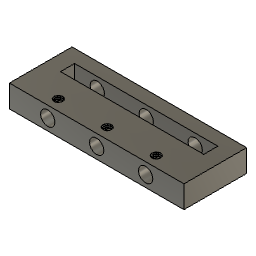
Cart Mount v2 (Autodesk Fusion 360 design; units mm, degrees)
Autodesk Fusion 360 part; units mm, degrees
sketch "Sketch1" plane through (0, 0, 0) normal (0, 1, 0) x (1, 0, 0)
  line L0 (39, 10) -> (-39, 10)
  line L1 (-39, 10) -> (-39, -10)
  line L2 (-39, -10) -> (39, -10)
  line L3 (39, -10) -> (39, 10)
  line L4 (39, 10) -> (-39, -10) construction
  line L5 (-39, 10) -> (39, -10) construction
  dimension "d1" = 78
  dimension "d2" = 20
  constraint horizontal L0
  constraint perpendicular L0 L1
  constraint parallel L0 L2
  constraint parallel L1 L3
  constraint coincident L4 origin
  constraint coincident L5 origin
  measures "d1" distance of L1.end L2.end
  measures "d2" distance of L0.end L1.end
extrude "Extrude1" add sketch "Sketch1" along normal mid plane 28 makes body 1
extrude "Extrude2" cut 1 faces at (-13, -4.6667, 10) along direction (0, 0, -1) blind 10 on bodies 1 bodies 1
sketch "Sketch2" plane through (0, -14, 0) normal (0, -1, 0) x (1, 0, 0)
  line L0 (39, 0) -> (-39, 0)
  line L1 (-39, 0) -> (-39, -10)
  line L2 (-39, -10) -> (39, -10)
  line L3 (39, -10) -> (39, 0)
  line L4 (0, 0) -> (0, -5)
  line L5 (0, -5) -> (21.875, -5)
  line L6 (0, -5) -> (-21.875, -5)
  dimension "d7" = 21.875
  dimension "d8" = 21.875
  constraint coincident L4.start origin
  constraint perpendicular L0 L4
  constraint perpendicular L4 L5
  constraint perpendicular L4 L6
  measures "d7" distance of L4.end L5.end
  measures "d8" distance of L4.end L6.end
hole "Hole1" at (-21.875, -14, -5) at (0, -14, -5) at (21.875, -14, -5) direction (0, 1, 0) diameter 6.4 depth 40.4 tip angle 118 bodies 1
sketch "Sketch3" plane through (0, 0, 0) normal (0, 0, 1) x (-1, 0, 0)
  line L0 (-39, 14) -> (-39, -14)
  line L1 (-39, -14) -> (39, -14)
  line L2 (39, -14) -> (39, 14)
  line L3 (39, 14) -> (-39, 14)
  line L4 (0, 14) -> (0, 9)
  line L5 (0, 9) -> (-21.875, 9)
  line L6 (0, 9) -> (21.875, 9)
  dimension "d12" = 21.875
  dimension "d13" = 21.875
  constraint midpoint L3 L4.start
  constraint perpendicular L3 L4
  constraint perpendicular L4 L5
  constraint perpendicular L4 L6
  measures "d12" distance of L4.end L5.end
  measures "d13" distance of L4.end L6.end
hole "Hole2" at (0, -9, 0) at (-21.875, -9, 0) at (21.875, -9, 0) direction (0, 0, -1) diameter 3.416 depth 4.4 tip angle 118 bodies 1
thread "Thread1" "ANSI Unified Screw Threads 0.164(#8) 8-32 UNC 2B" major diameter 4.1656 minor diameter 3.4163 pitch 0.7937 angle 60 modelled right hand crest width 0.2341 on face at (-1.708, -9.0099, -0.7646) crest through (1.7082, -9, -0.1984) on face at (-23.583, -9.0099, -0.7646) crest through (-20.1668, -9, -0.1984) on face at (20.167, -9.0099, -0.7646) crest through (23.5831, -9, -0.1984) on bodies 1
sketch "Sketch4" plane through (0, 0, 0) normal (0, 0, 1) x (-1, 0, 0)
  spline S0 degree 3 poles (1.0037, 10.825) (1.2209, 10.674) (1.4071, 10.4829) (1.6881, 10.048) (1.7836, 9.8108) (1.8744, 9.3235) (1.8728, 9.0789) (1.7889, 8.6765) (1.7315, 8.5168) (1.5758, 8.2237) (1.4795, 8.091) (1.3657, 7.9741) knots 0 0 0 0 0.079347 0.079347 0.155456 0.155456 0.228326 0.228326 0.279114 0.279114 0.328226 0.328226 0.328226 0.328226
  arc A0 (-1.3657, 7.9741) -> (1.3657, 7.9741) centre (0, 9) ccw
  spline S1 degree 3 poles (-1.3657, 7.9741) (-1.5233, 8.136) (-1.6469, 8.3277) (-1.8197, 8.7573) (-1.8634, 8.9926) (-1.8602, 9.4776) (-1.8092, 9.7228) (-1.6412, 10.1248) (-1.5443, 10.2864) (-1.3049, 10.5826) (-1.1624, 10.7147) (-1.0037, 10.825) knots 0 0 0 0 0.06777 0.06777 0.138771 0.138771 0.213001 0.213001 0.26909 0.26909 0.326867 0.326867 0.326867 0.326867
  arc A1 (1.0037, 10.825) -> (-1.0037, 10.825) centre (0, 9) ccw
  spline S2 degree 3 poles (22.8787, 10.825) (23.0959, 10.674) (23.2821, 10.4829) (23.5631, 10.048) (23.6586, 9.8108) (23.7494, 9.3235) (23.7478, 9.0789) (23.6639, 8.6765) (23.6065, 8.5168) (23.4508, 8.2237) (23.3545, 8.091) (23.2407, 7.9741) knots 0 0 0 0 0.079347 0.079347 0.155456 0.155456 0.228326 0.228326 0.279114 0.279114 0.328226 0.328226 0.328226 0.328226
  arc A2 (20.5093, 7.9741) -> (23.2407, 7.9741) centre (21.875, 9) ccw
  spline S3 degree 3 poles (20.5093, 7.9741) (20.3517, 8.136) (20.2281, 8.3277) (20.0553, 8.7573) (20.0116, 8.9926) (20.0148, 9.4776) (20.0658, 9.7228) (20.2338, 10.1248) (20.3307, 10.2864) (20.5701, 10.5826) (20.7126, 10.7147) (20.8713, 10.825) knots 0 0 0 0 0.06777 0.06777 0.138771 0.138771 0.213001 0.213001 0.26909 0.26909 0.326867 0.326867 0.326867 0.326867
  arc A3 (22.8787, 10.825) -> (20.8713, 10.825) centre (21.875, 9) ccw
  spline S4 degree 3 poles (-20.8713, 10.825) (-20.6541, 10.674) (-20.4679, 10.4829) (-20.1869, 10.048) (-20.0914, 9.8108) (-20.0006, 9.3235) (-20.0022, 9.0789) (-20.0861, 8.6765) (-20.1435, 8.5168) (-20.2992, 8.2237) (-20.3955, 8.091) (-20.5093, 7.9741) knots 0 0 0 0 0.079347 0.079347 0.155456 0.155456 0.228326 0.228326 0.279114 0.279114 0.328226 0.328226 0.328226 0.328226
  arc A4 (-23.2407, 7.9741) -> (-20.5093, 7.9741) centre (-21.875, 9) ccw
  spline S5 degree 3 poles (-23.2407, 7.9741) (-23.3983, 8.136) (-23.5219, 8.3277) (-23.6947, 8.7573) (-23.7384, 8.9926) (-23.7352, 9.4776) (-23.6842, 9.7228) (-23.5162, 10.1248) (-23.4193, 10.2864) (-23.1799, 10.5826) (-23.0374, 10.7147) (-22.8787, 10.825) knots 0 0 0 0 0.06777 0.06777 0.138771 0.138771 0.213001 0.213001 0.26909 0.26909 0.326867 0.326867 0.326867 0.326867
  arc A5 (-20.8713, 10.825) -> (-22.8787, 10.825) centre (-21.875, 9) ccw
  line L0 (-39, 14) -> (-39, -14)
  line L1 (-39, -14) -> (39, -14)
  line L2 (39, -14) -> (39, 14)
  line L3 (39, 14) -> (-39, 14)
  line L4 (-32, -8.15) -> (32, -8.15)
  line L5 (32, -8.15) -> (32, -1.85)
  line L6 (32, -1.85) -> (-32, -1.85)
  line L7 (-32, -1.85) -> (-32, -8.15)
  line L8 (-32, -8.15) -> (32, -1.85) construction
  line L9 (32, -8.15) -> (-32, -1.85) construction
  point P0 (0, -5)
  dimension "d17" = 6.3
  constraint horizontal L4
  constraint perpendicular L4 L5
  constraint parallel L4 L6
  constraint parallel L5 L7
  constraint coincident L8 P0
  constraint coincident L9 P0
  measures "d17" distance of L4.end L5.end
extrude "Extrude3" cut sketch "Sketch4" against normal blind 10 contours L4 L5 L6 L7 bodies 1
copy_body "Body->Comp1" bodies 1 removing the originals makes body 2 in component "Component"
component "Component" placed x (1, 0, 0) y (0, 1, 0) z (0, 0, 1) at (0, 0, 0)
